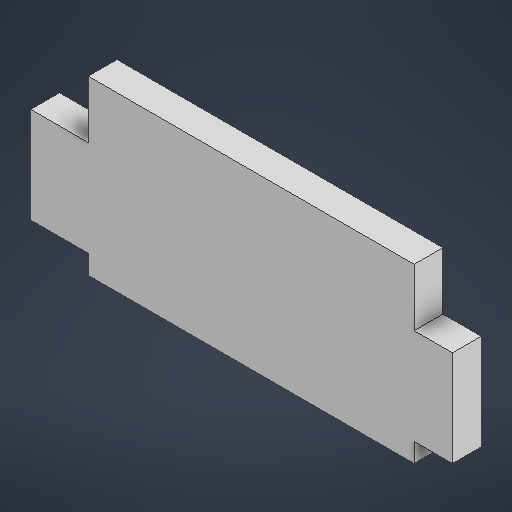
# Autodesk Inventor part: Frontrail
Saved by Autodesk Inventor 2027 (Build 310192000, 192)
## iProperties
Created: 2026-05-13
Part Number: Frontrail
Material: Generic
Document SubType Name: Modeling
Designer: alexy
Density: 1 g/cm^3
Appearance: Default
Author: alexy
Autodesk Inventor part; units mm, degrees
ref_plane "YZ Plane" through (0, 0, 0) normal (1, 0, 0) x (0, 1, 0)
ref_plane "XZ Plane" through (0, 0, 0) normal (0, 1, 0) x (-1, 0, 0)
ref_plane "XY Plane" through (0, 0, 0) normal (0, 0, 1) x (1, 0, 0)
sketch "Sketch1" plane through (0, 0, 0) normal (0, 0, 1) x (1, 0, 0)
  line L0 (0, 0) -> (34, 0)
  line L1 (34, 0) -> (34, 18)
  line L2 (34, 18) -> (0, 18)
  line L3 (0, 18) -> (0, 0)
  line L4 (-6, 12) -> (0, 12)
  line L5 (0, 12) -> (0, 2)
  line L6 (0, 2) -> (-6, 2)
  line L7 (-6, 2) -> (-6, 12)
  line L8 (-6, 12) -> (0, 2) construction
  line L9 (0, 12) -> (-6, 2) construction
  line L10 (38, 12) -> (34, 12)
  line L11 (34, 12) -> (34, 2)
  line L12 (34, 2) -> (38, 2)
  line L13 (38, 2) -> (38, 12)
  line L14 (38, 12) -> (34, 2) construction
  line L15 (34, 12) -> (38, 2) construction
  point P0 (-3, 7)
  point P1 (36, 7)
  point P2 (34, 12)
  point P3 (0, 12)
  dimension "d0" = 34
  dimension "d2" = 4
  dimension "d3" = 6
  dimension "d4" = 10
  dimension "d5" = 10
  dimension "d8" = 2
  dimension "d9" = 6
  constraints: 32 end point, 6 parallel, 4 midpoint, 3 horizontal, 3 perpendicular, 2 point on line, 1 horizontal alignment
  measures "d0" distance of L1.end L2.end
  measures "d2" distance of L10.start L10.end
  measures "d3" distance of L4.start L4.end
  measures "d4" distance of L6.end L4.start
  measures "d5" distance of L12.end L10.start
  measures "d8" distance of L0.start L5.end
  measures "d9" distance of L4.end L2.end
extrude "Extrusion1" add sketch "Sketch1" along normal blind 3
body "Solid1"
